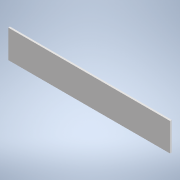
# Autodesk Inventor part: mounting plate
Saved by Autodesk Inventor 2020 (Build 240168000, 168)
## iProperties
Created: 2021-02-27
Part Number: mounting plate
Material: Generic
Document SubType Name: Modeling
Designer: Bernard Li
Density: 1 g/cm^3
Appearance: Default
Author: Bernard Li
Autodesk Inventor part; units mm, degrees
ref_plane "YZ Plane" through (0, 0, 0) normal (1, 0, 0) x (0, 1, 0)
ref_plane "XZ Plane" through (0, 0, 0) normal (0, 1, 0) x (-1, 0, 0)
ref_plane "XY Plane" through (0, 0, 0) normal (0, 0, 1) x (1, 0, 0)
sketch "Sketch1" plane through (0, 0, 0) normal (0, 0, 1) x (1, 0, 0)
  line L0 (0, 0) -> (0, -101.6)
  line L1 (0, -101.6) -> (584.2, -101.6)
  line L2 (584.2, -101.6) -> (584.2, 0)
  line L3 (584.2, 0) -> (0, 0)
  dimension "d0" = 101.6
  dimension "d1" = 584.2
  constraints: 8 end point, 2 parallel, 1 perpendicular, 1 vertical
  measures "d0" distance of L0.start L0.end
  measures "d1" distance of L2.end L0.start
extrude "Extrusion1" add sketch "Sketch1" along normal blind 6.35
body "Solid1"
